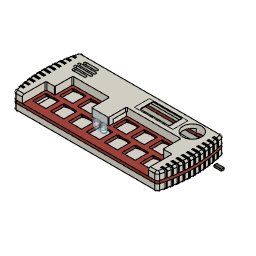
pianissimo_retro_case (Autodesk Fusion 360 design; units mm, degrees)
Autodesk Fusion 360 part; units mm, degrees
(part 1 of 2)
sketch "acrylic_import" plane through (0, 0, 0) normal (0, 0, 1) x (1, 0, 0)
  line L0 (-9.525, 176.95625) -> (51.15, 176.95625)
  line L1 (51.15, 171.95625) -> (51.15, 176.95625)
  line L2 (21.5, 189.35) -> (35.65, 189.35)
  line L3 (63.15, 171.95625) -> (63.15, 176.95625)
  line L4 (116.75, 189.35) -> (130.9, 189.35)
  line L5 (63.15, 171.95625) -> (133.875, 171.95625)
  circle A0 centre (-5.025, 185.875) radius 1.5
  line L6 (63.15, 176.95625) -> (142.875, 176.95625)
  circle A1 centre (-5.025, 172.45625) radius 1.5
  line L7 (133.875, 171.95625) -> (133.875, 111.375)
  line L8 (-0.525, 111.375) -> (133.875, 111.375)
  line L9 (-9.525, 101.95625) -> (-9.525, 31.375)
  circle A2 centre (-5.025, 35.875) radius 1.5
  circle A3 centre (138.375, 185.875) radius 1.5
  line L10 (-9.525, 106.375) -> (142.875, 106.375)
  line L11 (142.875, 101.95625) -> (142.875, 31.375)
  line L12 (59.6, 189.35) -> (73.75, 189.35)
  line L13 (142.875, 106.375) -> (142.875, 176.95625)
  line L14 (-9.525, 176.95625) -> (-9.525, 106.375)
  circle A4 centre (-5.025, 97.45625) radius 1.5
  line L15 (40.55, 189.35) -> (54.7, 189.35)
  line L16 (142.875, -43.625) -> (142.875, 26.95625)
  line L17 (35.65, 189.35) -> (35.65, 203.5)
  circle A5 centre (138.375, 172.45625) radius 1.5
  line L18 (63.15, 96.95625) -> (63.15, 101.95625)
  line L19 (2.45, 189.35) -> (16.6, 189.35)
  line L20 (-0.525, 111.375) -> (-0.525, 171.95625)
  line L21 (97.7, 189.35) -> (111.85, 189.35)
  line L22 (-0.525, 171.95625) -> (51.15, 171.95625)
  circle A6 centre (138.375, 110.875) radius 1.5
  line L23 (142.875, 101.95625) -> (63.15, 101.95625)
  circle A7 centre (-5.025, -39.125) radius 1
  circle A8 centre (-5.025, 22.45625) radius 1
  line L24 (-9.525, 251.95625) -> (-9.525, 181.375)
  line L25 (-9.525, 181.375) -> (142.875, 181.375)
  circle A9 centre (-5.025, 110.875) radius 1.5
  line L26 (78.65, 189.35) -> (92.8, 189.35)
  line L27 (-9.525, -43.625) -> (142.875, -43.625)
  line L28 (111.85, 189.35) -> (111.85, 203.5)
  line L29 (78.65, 203.5) -> (78.65, 189.35)
  circle A10 centre (138.375, 22.45625) radius 1
  line L30 (-9.525, 26.95625) -> (142.875, 26.95625)
  circle A11 centre (138.375, 97.45625) radius 1.5
  line L31 (133.875, 36.375) -> (133.875, 96.95625)
  line L32 (51.15, 96.95625) -> (51.15, 101.95625)
  line L33 (59.6, 203.5) -> (59.6, 189.35)
  line L34 (-9.525, 101.95625) -> (51.15, 101.95625)
  circle A12 centre (138.375, -39.125) radius 1
  line L35 (-9.525, 26.95625) -> (-9.525, -43.625)
  line L36 (-0.525, 36.375) -> (133.875, 36.375)
  line L37 (51.15, 96.95625) -> (-0.525, 96.95625)
  line L38 (-9.525, 31.375) -> (142.875, 31.375)
  circle A13 centre (138.375, 35.875) radius 1.5
  line L39 (-0.525, 96.95625) -> (-0.525, 36.375)
  line L40 (63.15, 96.95625) -> (133.875, 96.95625)
  arc A14 (120.930314, 228.525) -> (126.719686, 228.525) centre (123.825, 238.096875) ccw
  arc A15 (128.463046, 246.95625) -> (119.186954, 246.95625) centre (123.825, 238.096875) ccw
  line L41 (88.175, 208.4) -> (102.325, 208.4)
  line L42 (16.6, 189.35) -> (16.6, 203.5)
  line L43 (63.15, 246.95625) -> (63.15, 251.95625)
  line L44 (83.275, 208.4) -> (83.275, 222.55)
  circle A16 centre (138.375, 247.45625) radius 1.5
  line L45 (111.85, 203.5) -> (97.7, 203.5)
  circle A17 centre (138.375, 260.875) radius 1.5
  line L46 (2.45, 203.5) -> (2.45, 189.35)
  line L47 (133.875, 228.525) -> (133.875, 246.95625)
  line L48 (102.325, 208.4) -> (102.325, 222.55)
  line L49 (69.125, 208.4) -> (83.275, 208.4)
  line L50 (63.15, 251.95625) -> (142.875, 251.95625)
  line L51 (133.875, 228.525) -> (126.719686, 228.525)
  line L52 (130.9, 203.5) -> (116.75, 203.5)
  line L53 (92.8, 203.5) -> (78.65, 203.5)
  line L54 (102.325, 222.55) -> (88.175, 222.55)
  line L55 (83.275, 222.55) -> (69.125, 222.55)
  line L56 (121.375, 208.4) -> (121.375, 222.55)
  line L57 (121.375, 222.55) -> (107.225, 222.55)
  line L58 (107.225, 208.4) -> (121.375, 208.4)
  line L59 (69.125, 222.55) -> (69.125, 208.4)
  line L60 (88.175, 222.55) -> (88.175, 208.4)
  line L61 (107.225, 222.55) -> (107.225, 208.4)
  arc A18 (3.381227, 395.390581) -> (3.386093, 392.890586) centre (3.38366, 394.140584) ccw
  line L62 (9, 281.475) -> (9, 300.525)
  arc A19 (15.876065, 392.914896) -> (15.871199, 395.414891) centre (15.873632, 394.164893) ccw
  line L63 (9, 375.525) -> (48.15, 375.525)
  line L64 (-9.525, 401.95625) -> (-9.525, 331.375)
  line L65 (15.876065, 392.914896) -> (3.386093, 392.890586)
  line L66 (9, 356.475) -> (9, 375.525)
  line L67 (-0.525, 281.475) -> (9, 281.475)
  line L68 (48.15, 300.525) -> (48.15, 303.525)
  line L69 (1.169417, 391.395696) -> (18.021701, 391.414893)
  line L70 (-0.525, 331.375) -> (-0.525, 356.475)
  circle A20 centre (-5.025, 335.875) radius 1
  circle A21 centre (-5.025, 322.45625) radius 1.5
  circle A22 centre (-5.025, 397.45625) radius 1
  arc A23 (18.024549, 388.914894) -> (18.021701, 391.414893) centre (18.023125, 390.164893) ccw
  arc A24 (18.024544, 384.914894) -> (18.021707, 387.414893) centre (18.023125, 386.164893) ccw
  line L71 (15.877503, 380.914899) -> (3.387616, 380.876226)
  line L72 (18.024544, 384.914894) -> (1.172264, 384.895769)
  line L73 (-9.525, 331.375) -> (-0.525, 331.375)
  line L74 (48.15, 356.475) -> (48.15, 375.525)
  line L75 (3.379875, 383.376214) -> (15.869762, 383.414887)
  line L76 (3.381227, 395.390581) -> (15.871199, 395.414891)
  arc A25 (1.169417, 391.395696) -> (1.172265, 388.895698) centre (1.170841, 390.145697) ccw
  line L77 (133.875, 356.475) -> (133.875, 331.375)
  line L78 (133.875, 356.475) -> (124.35, 356.475)
  line L79 (1.169426, 387.395767) -> (18.021707, 387.414893)
  line L80 (9, 300.525) -> (48.15, 300.525)
  line L81 (48.15, 303.525) -> (-0.525, 303.525)
  arc A26 (15.877503, 380.914899) -> (15.869762, 383.414887) centre (15.873632, 382.164893) ccw
  line L82 (18.024549, 388.914894) -> (1.172265, 388.895698)
  arc A27 (3.379875, 383.376214) -> (3.387616, 380.876226) centre (3.383745, 382.12622) ccw
  line L83 (48.15, 211.475) -> (48.15, 225.525)
  line L84 (97.7, 203.5) -> (97.7, 189.35)
  circle A28 centre (-5.025, 260.875) radius 1.5
  arc A29 (142.875, 181.375) -> (142.875, 251.95625) centre (20.832179, 216.665625) ccw
  line L85 (63.15, 246.95625) -> (119.186954, 246.95625)
  line L86 (66.15, 225.525) -> (66.15, 211.475)
  line L87 (66.15, 225.525) -> (66.15, 228.525)
  line L88 (120.930314, 228.525) -> (66.15, 228.525)
  line L89 (73.75, 189.35) -> (73.75, 203.5)
  line L90 (40.55, 203.5) -> (40.55, 189.35)
  line L91 (54.7, 189.35) -> (54.7, 203.5)
  line L92 (128.463046, 246.95625) -> (133.875, 246.95625)
  line L93 (133.875, 256.375) -> (142.875, 256.375)
  line L94 (54.7, 203.5) -> (40.55, 203.5)
  line L95 (-0.525, 246.95625) -> (51.15, 246.95625)
  line L96 (119.186954, 321.95625) -> (-0.525, 321.95625)
  line L97 (66.15, 211.475) -> (48.15, 211.475)
  line L98 (73.75, 203.5) -> (59.6, 203.5)
  line L99 (-0.525, 246.95625) -> (-0.525, 228.525)
  line L100 (-9.525, 251.95625) -> (51.15, 251.95625)
  circle A30 centre (-5.025, 247.45625) radius 1.5
  line L101 (133.875, 281.475) -> (133.875, 256.375)
  line L102 (45.175, 208.4) -> (45.175, 222.55)
  line L103 (142.875, 256.375) -> (142.875, 326.95625)
  line L104 (26.125, 222.55) -> (11.975, 222.55)
  line L105 (11.975, 208.4) -> (26.125, 208.4)
  line L106 (35.65, 203.5) -> (21.5, 203.5)
  arc A31 (-9.525, 251.95625) -> (-9.525, 181.375) centre (112.517821, 216.665625) ccw
  line L107 (130.9, 189.35) -> (130.9, 203.5)
  line L108 (116.75, 203.5) -> (116.75, 189.35)
  line L109 (-9.525, 326.95625) -> (-9.525, 256.375)
  line L110 (31.025, 222.55) -> (31.025, 208.4)
  line L111 (66.15, 356.475) -> (48.15, 356.475)
  line L112 (21.5, 203.5) -> (21.5, 189.35)
  line L113 (142.875, 181.375) -> (142.875, 251.95625)
  line L114 (-9.525, 256.375) -> (-0.525, 256.375)
  line L115 (-0.525, 256.375) -> (-0.525, 281.475)
  line L116 (51.15, 246.95625) -> (51.15, 251.95625)
  line L117 (-9.525, 326.95625) -> (142.875, 326.95625)
  line L118 (45.175, 222.55) -> (31.025, 222.55)
  line L119 (92.8, 189.35) -> (92.8, 203.5)
  line L120 (16.6, 203.5) -> (2.45, 203.5)
  line L121 (11.975, 222.55) -> (11.975, 208.4)
  line L122 (26.125, 208.4) -> (26.125, 222.55)
  line L123 (31.025, 208.4) -> (45.175, 208.4)
  circle A32 centre (138.375, 397.45625) radius 1
  line L124 (48.15, 228.525) -> (-0.525, 228.525)
  line L125 (124.35, 375.525) -> (66.15, 375.525)
  line L126 (142.875, 331.375) -> (142.875, 401.95625)
  line L127 (124.35, 356.475) -> (124.35, 375.525)
  line L128 (133.875, 331.375) -> (142.875, 331.375)
  line L129 (-9.525, 401.95625) -> (142.875, 401.95625)
  line L130 (-0.525, 356.475) -> (9, 356.475)
  line L131 (66.15, 300.525) -> (66.15, 303.525)
  line L132 (128.463046, 321.95625) -> (133.875, 321.95625)
  circle A33 centre (138.375, 322.45625) radius 1.5
  line L133 (66.15, 375.525) -> (66.15, 356.475)
  line L134 (124.35, 281.475) -> (124.35, 300.525)
  line L135 (48.15, 225.525) -> (48.15, 228.525)
  line L136 (133.875, 303.525) -> (133.875, 321.95625)
  line L137 (133.875, 281.475) -> (124.35, 281.475)
  line L138 (133.875, 303.525) -> (126.719686, 303.525)
  line L139 (-0.525, 321.95625) -> (-0.525, 303.525)
  line L140 (120.930314, 303.525) -> (66.15, 303.525)
  circle A34 centre (138.375, 335.875) radius 1
  arc A35 (1.169426, 387.395767) -> (1.172264, 384.895768) centre (1.170845, 386.145768) ccw
  arc A36 (128.463046, 321.95625) -> (119.186954, 321.95625) centre (123.825, 313.096875) ccw
  circle A37 centre (123.825, 388.096875) radius 10
  line L141 (124.35, 300.525) -> (66.15, 300.525)
  arc A38 (120.930314, 303.525) -> (126.719686, 303.525) centre (123.825, 313.096875) ccw
  point P0 (-5.025, 172.45625)
  dimension "d157" = 2
  dimension "d158" = 2
  dimension "d159" = 2
  dimension "d160" = 2
  dimension "d161" = 3
  dimension "d162" = 3
  dimension "d163" = 3
  dimension "d164" = 3
  dimension "d165" = 3
  dimension "d166" = 3
  dimension "d167" = 3
  dimension "d168" = 3
  dimension "d169" = 3
  dimension "d170" = 3
  dimension "d171" = 3
  dimension "d172" = 3
  dimension "d173" = 3
  dimension "d174" = 3
  dimension "d175" = 3
  dimension "d176" = 2
  dimension "d177" = 2
  dimension "d178" = 2
  dimension "d179" = 2
  dimension "d180" = 3
  dimension "d181" = 20
  dimension "d182" = 2.5
  dimension "d183" = 2.5
  dimension "d184" = 2.5
  dimension "d185" = 2.5
  dimension "d186" = 2.5
  dimension "d187" = 2.5
  dimension "d188" = 2.5
  dimension "d189" = 2.5
  dimension "d190" = 20
  dimension "d191" = 20
  constraint perpendicular L51 L99
  constraint coincident L124.start L51
  constraint perpendicular L51 L135
  constraint perpendicular L51 L87
  constraint perpendicular L47 L95
  constraint perpendicular L138 L139
  constraint coincident L68.end L138
  constraint perpendicular L68 L138
  constraint perpendicular L131 L138
  constraint coincident L93.start L114
  constraint perpendicular L111 L133
  constraint coincident L77.end L73
  constraint collinear L0 L6
  constraint collinear L5 L22
  constraint collinear L50 L100
  constraint collinear L85 L95
  constraint collinear L51 L124
  constraint collinear L93 L114
  constraint collinear L81 L138
  constraint collinear L73 L128
  constraint perpendicular L27 L35
  constraint perpendicular L16 L30
  constraint perpendicular L64 L73
  constraint perpendicular L70 L130
  constraint perpendicular L126 L129
  constraint perpendicular L77 L128
  constraint perpendicular L109 L114
  constraint perpendicular L67 L115
  constraint perpendicular L93 L101
  constraint perpendicular L24 L25
  constraint perpendicular L25 L113
  constraint perpendicular L10 L14
  constraint perpendicular L6 L13
  constraint perpendicular L7 L8
  constraint perpendicular L20 L22
  constraint perpendicular L36 L39
  constraint perpendicular L9 L38
  constraint tangent A18 L76
  constraint tangent A19 L76
  constraint tangent A19 L65
  constraint tangent A18 L65
  constraint tangent L69 A25
  constraint tangent L69 A23
  constraint tangent A23 L82
  constraint tangent A25 L82
  constraint tangent L79 A35
  constraint tangent A24 L79
  constraint tangent A24 L72
  constraint tangent L72 A35
  constraint tangent L75 A27
  constraint tangent L75 A26
  constraint tangent L71 A26
  constraint tangent L71 A27
  constraint collinear L85 L92
  constraint collinear L51 L88
  constraint concentric A14 A15
  constraint collinear L138 L140
  constraint concentric A36 A38
  constraint perpendicular L103 L117
  constraint perpendicular L96 L139
  constraint perpendicular L32 L34
  constraint perpendicular L37 L39
  constraint perpendicular L31 L40
  constraint perpendicular L18 L23
  measures "d157" diameter of A7
  measures "d158" diameter of A8
  measures "d159" diameter of A10
  measures "d160" diameter of A12
  measures "d161" diameter of A2
  measures "d162" diameter of A4
  measures "d163" diameter of A11
  measures "d164" diameter of A13
  measures "d165" diameter of A9
  measures "d166" diameter of A5
  measures "d167" diameter of A6
  measures "d168" diameter of A0
  measures "d169" diameter of A30
  measures "d170" diameter of A16
  measures "d171" diameter of A3
  measures "d172" diameter of A1
  measures "d173" diameter of A28
  measures "d174" diameter of A33
  measures "d175" diameter of A17
  measures "d176" diameter of A20
  measures "d177" diameter of A22
  measures "d178" diameter of A32
  measures "d179" diameter of A34
  measures "d180" diameter of A21
  measures "d181" diameter of A37
  measures "d182" diameter of A19
  measures "d183" diameter of A23
  measures "d184" diameter of A24
  measures "d185" diameter of A26
  measures "d186" diameter of A27
  measures "d187" diameter of A35
  measures "d188" diameter of A25
  measures "d189" diameter of A18
  measures "d190" diameter of A36
  measures "d191" diameter of A15
sketch "plate" plane through (0, 0, 0) normal (0, 0, 1) x (1, 0, 0)
  line L0 (111.85, -21.5) -> (97.7, -21.5)
  line L1 (121.375, -2.45) -> (107.225, -2.45)
  line L2 (88.175, -16.6) -> (102.325, -16.6)
  line L3 (83.275, -16.6) -> (83.275, -2.45)
  line L4 (102.325, -16.6) -> (102.325, -2.45)
  line L5 (83.275, -2.45) -> (69.125, -2.45)
  line L6 (130.9, -21.5) -> (116.75, -21.5)
  line L7 (69.125, -2.45) -> (69.125, -16.6)
  line L8 (107.225, -2.45) -> (107.225, -16.6)
  line L9 (88.175, -2.45) -> (88.175, -16.6)
  line L10 (102.325, -2.45) -> (88.175, -2.45)
  line L11 (121.375, -16.6) -> (121.375, -2.45)
  line L12 (92.8, -21.5) -> (78.65, -21.5)
  line L13 (120.930314, 3.525) -> (66.65, 3.525)
  line L14 (92.8, -35.65) -> (92.8, -21.5)
  line L15 (130.9, -35.65) -> (130.9, -21.5)
  line L16 (73.75, -35.65) -> (73.75, -21.5)
  line L17 (63.15, 21.95625) -> (63.15, 26.95625)
  line L18 (128.463046, 21.95625) -> (133.875, 21.95625)
  line L19 (116.75, -21.5) -> (116.75, -35.65)
  arc A0 (128.463046, 21.95625) -> (119.186954, 21.95625) centre (123.825, 13.096875) ccw
  line L20 (66.65, 0.525) -> (66.65, -13.525)
  line L21 (69.125, -16.6) -> (83.275, -16.6)
  line L22 (16.6, -35.65) -> (16.6, -21.5)
  line L23 (107.225, -16.6) -> (121.375, -16.6)
  line L24 (142.875, -43.625) -> (142.875, 26.95625)
  line L25 (-9.525, 26.95625) -> (-9.525, -43.625)
  line L26 (63.15, 21.95625) -> (119.186954, 21.95625)
  line L27 (97.7, -21.5) -> (97.7, -35.772243)
  line L28 (133.875, 3.525) -> (126.719686, 3.525)
  line L29 (133.875, 3.525) -> (133.875, 21.95625)
  arc A1 (120.930314, 3.525) -> (126.719686, 3.525) centre (123.825, 13.096875) ccw
  line L30 (21.5, -21.5) -> (21.5, -35.65)
  line L31 (63.15, 26.95625) -> (142.875, 26.95625)
  line L32 (111.85, -35.772243) -> (111.85, -21.5)
  line L33 (35.65, -35.65) -> (35.65, -21.5)
  circle A2 centre (138.375, 22.45625) radius 1.05
  line L34 (66.65, 0.525) -> (66.65, 3.525)
  line L35 (54.7, -35.65) -> (54.7, -21.5)
  line L36 (26.125, -2.45) -> (11.975, -2.45)
  line L37 (97.7, -35.772243) -> (111.85, -35.772243)
  line L38 (40.55, -21.5) -> (40.55, -35.65)
  line L39 (-9.525, 26.95625) -> (51.15, 26.95625)
  line L40 (31.025, -16.6) -> (45.175, -16.6)
  line L41 (78.65, -21.5) -> (78.65, -35.65)
  line L42 (59.6, -21.5) -> (59.6, -35.65)
  line L43 (47.65, 3.525) -> (-0.525, 3.525)
  line L44 (47.65, -13.525) -> (47.65, 0.525)
  line L45 (40.55, -35.65) -> (54.7, -35.65)
  line L46 (45.175, -2.45) -> (31.025, -2.45)
  arc A3 (-9.525, 26.95625) -> (-9.525, -43.625) centre (112.517821, -8.334375) ccw
  circle A4 centre (-5.025, -39.125) radius 1.05
  line L47 (-9.525, -43.625) -> (142.875, -43.625)
  line L48 (16.6, -21.5) -> (2.45, -21.5)
  line L49 (-0.525, 21.95625) -> (51.15, 21.95625)
  line L50 (35.65, -21.5) -> (21.5, -21.5)
  line L51 (-0.525, 21.95625) -> (-0.525, 3.525)
  circle A5 centre (-5.025, 22.45625) radius 1.05
  line L52 (73.75, -21.5) -> (59.6, -21.5)
  line L53 (31.025, -2.45) -> (31.025, -16.6)
  arc A6 (142.875, -43.625) -> (142.875, 26.95625) centre (20.832179, -8.334375) ccw
  line L54 (47.65, 0.525) -> (47.65, 3.525)
  line L55 (21.5, -35.65) -> (35.65, -35.65)
  line L56 (11.975, -2.45) -> (11.975, -16.6)
  line L57 (11.975, -16.6) -> (26.125, -16.6)
  line L58 (116.75, -35.65) -> (130.9, -35.65)
  line L59 (78.65, -35.65) -> (92.8, -35.65)
  line L60 (26.125, -16.6) -> (26.125, -2.45)
  line L61 (66.65, -13.525) -> (47.65, -13.525)
  line L62 (54.7, -21.5) -> (40.55, -21.5)
  line L63 (51.15, 21.95625) -> (51.15, 26.95625)
  line L64 (59.6, -35.65) -> (73.75, -35.65)
  circle A7 centre (138.375, -39.125) radius 1.05
  line L65 (45.175, -16.6) -> (45.175, -2.45)
  line L66 (2.45, -21.5) -> (2.45, -35.65)
  line L67 (2.45, -35.65) -> (16.6, -35.65)
  line L68 (51.15, 26.95625) -> (63.15, 26.95625)
  line L69 (63.15, 21.95625) -> (51.15, 21.95625)
  line L70 (46.15, 23.95625) -> (46.15, 24.95625)
  line L71 (41.65, 23.95625) -> (41.65, 24.95625)
  line L72 (68.15, 23.95625) -> (68.15, 24.95625)
  line L73 (72.65, 23.95625) -> (72.65, 24.95625)
  line L74 (42.15, 25.45625) -> (45.65, 25.45625)
  line L75 (42.15, 23.45625) -> (45.65, 23.45625)
  line L76 (68.65, 25.45625) -> (72.15, 25.45625)
  line L77 (68.65, 23.45625) -> (72.15, 23.45625)
  arc A8 (42.15, 25.45625) -> (41.65, 24.95625) centre (42.15, 24.95625) ccw
  arc A9 (41.65, 23.95625) -> (42.15, 23.45625) centre (42.15, 23.95625) ccw
  arc A10 (45.65, 23.45625) -> (46.15, 23.95625) centre (45.65, 23.95625) ccw
  arc A11 (46.15, 24.95625) -> (45.65, 25.45625) centre (45.65, 24.95625) ccw
  arc A12 (68.65, 25.45625) -> (68.15, 24.95625) centre (68.65, 24.95625) ccw
  arc A13 (72.65, 24.95625) -> (72.15, 25.45625) centre (72.15, 24.95625) ccw
  arc A14 (72.15, 23.45625) -> (72.65, 23.95625) centre (72.15, 23.95625) ccw
  arc A15 (68.15, 23.95625) -> (68.65, 23.45625) centre (68.65, 23.95625) ccw
  line L78 (160.000002, 0) -> (168.000002, 0)
  line L79 (168.000002, 0) -> (168.000002, 3)
  line L80 (168.000002, 3) -> (160.000002, 3)
  line L81 (160.000002, 3) -> (160.000002, 0)
  dimension "d36" = 2.1
  dimension "d37" = 2.1
  dimension "d38" = 2.1
  dimension "d39" = 2.1
  dimension "d40" = 20
  dimension "d216" = 0.5
  dimension "d220" = 8
  dimension "d221" = 3
  constraint perpendicular L28 L51
  constraint coincident L43.start L28
  constraint perpendicular L28 L54
  constraint perpendicular L28 L34
  constraint perpendicular L29 L49
  constraint collinear L31 L39
  constraint collinear L26 L49
  constraint collinear L28 L43
  constraint perpendicular L25 L47
  constraint perpendicular L24 L47
  constraint collinear L18 L26
  constraint collinear L13 L28
  constraint concentric A0 A1
  constraint perpendicular L17 L68
  constraint perpendicular L63 L69
  constraint tangent L76 A12
  constraint tangent L72 A12
  constraint tangent L76 A13
  constraint tangent L77 A14
  constraint tangent L77 A15
  constraint tangent L72 A15
  constraint horizontal L78
  constraint vertical L79
  constraint horizontal L80
  constraint vertical L81
  measures "d36" diameter of A4
  measures "d37" diameter of A5
  measures "d38" diameter of A2
  measures "d39" diameter of A7
  measures "d40" diameter of A0
  measures "d216" radius of A8
sketch "bottom" plane through (0, 0, 0) normal (0, 0, 1) x (1, 0, 0)
  line L0 (-9.525, 26.95625) -> (-9.525, -43.625)
  line L1 (-9.525, -43.625) -> (142.875, -43.625)
  circle A0 centre (138.375, 22.45625) radius 2.5
  circle A1 centre (-5.025, 22.45625) radius 2.5
  line L2 (-0.525, -38.625) -> (133.875, -38.625)
  circle A2 centre (-5.025, -39.125) radius 2.5
  line L3 (133.875, -38.625) -> (133.875, 21.95625)
  circle A3 centre (138.375, -39.125) radius 2.5
  line L4 (51.15, 21.95625) -> (51.15, 26.95625)
  line L5 (142.875, 26.95625) -> (142.875, -43.625)
  line L6 (-0.525, 21.95625) -> (-0.525, -38.625)
  line L7 (63.15, 21.95625) -> (63.15, 26.95625)
  arc A4 (142.875, -43.625) -> (142.875, 26.95625) centre (20.832179, -8.334375) ccw
  arc A5 (-9.525, 26.95625) -> (-9.525, -43.625) centre (112.517821, -8.334375) ccw
  line L8 (-0.525, 21.95625) -> (133.875, 21.95625)
  line L9 (-9.525, 26.95625) -> (142.875, 26.95625)
  circle A6 centre (-5.025, 22.45625) radius 1.05
  circle A7 centre (138.375, 22.45625) radius 1.05
  circle A8 centre (138.375, -39.125) radius 1.05
  circle A9 centre (-5.025, -39.125) radius 1.05
  dimension "d41" = 5
  dimension "d42" = 5
  dimension "d43" = 5
  dimension "d44" = 5
  dimension "d195" = 2.1
  dimension "d196" = 2.1
  dimension "d197" = 2.1
  dimension "d198" = 2.1
  constraint perpendicular L2 L6
  constraint perpendicular L0 L1
  constraint perpendicular L3 L8
  constraint perpendicular L0 L9
  constraint concentric A1 A6
  constraint concentric A0 A7
  constraint concentric A3 A8
  constraint concentric A2 A9
  measures "d41" diameter of A2
  measures "d42" diameter of A1
  measures "d43" diameter of A0
  measures "d44" diameter of A3
  measures "d195" diameter of A6
  measures "d196" diameter of A7
  measures "d197" diameter of A8
  measures "d198" diameter of A9
sketch "top" plane through (0, 0, 0) normal (0, 0, 1) x (1, 0, 0)
  line L0 (133.875, -43.625) -> (142.875, -43.625)
  line L1 (124.35, 0.525) -> (66.15, 0.525)
  line L2 (124.35, -18.525) -> (124.35, 0.525)
  line L3 (66.15, 0.525) -> (66.15, -18.525)
  line L4 (133.875, -18.525) -> (133.875, -43.625)
  line L5 (48.15, -18.525) -> (48.15, 0.525)
  line L6 (-9.525, 26.95625) -> (142.875, 26.95625)
  circle A0 centre (138.375, 22.45625) radius 1.5
  line L7 (-9.525, 26.95625) -> (-9.525, -43.625)
  line L8 (66.15, -18.525) -> (48.15, -18.525)
  line L9 (133.875, -18.525) -> (124.35, -18.525)
  circle A1 centre (-5.025, -39.125) radius 1.5
  line L10 (142.875, -43.625) -> (142.875, 26.95625)
  circle A2 centre (138.375, -39.125) radius 1.5
  circle A3 centre (-5.025, 22.45625) radius 1.5
  line L11 (9, -18.525) -> (9, 0.525)
  line L12 (-0.525, -43.625) -> (-0.525, -18.525)
  line L13 (-0.525, -18.525) -> (9, -18.525)
  line L14 (9, 0.525) -> (48.15, 0.525)
  line L15 (-9.525, -43.625) -> (-0.525, -43.625)
  line L16 (48.15, 3.525) -> (-0.525, 3.525)
  line L17 (48.15, 0.525) -> (48.15, 3.525)
  line L18 (66.15, 0.525) -> (66.15, 3.525)
  line L19 (66.15, 3.525) -> (133.875, 3.525)
  line L20 (133.875, 3.525) -> (133.875, 21.95625)
  line L21 (-0.525, 21.95625) -> (133.875, 21.95625)
  line L22 (-0.525, 21.95625) -> (-0.525, 3.525)
  arc A4 (-9.525, 26.95625) -> (-9.525, -43.625) centre (112.517821, -8.334375) ccw
  arc A5 (142.875, -43.625) -> (142.875, 26.95625) centre (20.832179, -8.334375) ccw
  line L23 (66.15, -13.525) -> (48.15, -13.525)
  dimension "d49" = 3
  dimension "d50" = 3
  dimension "d51" = 3
  dimension "d56" = 3
  constraint perpendicular L3 L8
  constraint coincident L0.start L15
  constraint collinear L0 L15
  constraint perpendicular L7 L15
  constraint perpendicular L12 L13
  constraint perpendicular L6 L10
  constraint perpendicular L0 L4
  constraint perpendicular L19 L20
  constraint perpendicular L20 L21
  measures "d49" diameter of A1
  measures "d50" diameter of A0
  measures "d51" diameter of A2
  measures "d56" diameter of A3
sketch "top_holes" plane through (0, 0, 0) normal (0, 0, 1) x (1, 0, 0)
  arc A0 (3.379875, 8.376214) -> (3.387616, 5.876226) centre (3.383745, 7.12622) ccw
  line L0 (3.379875, 8.376214) -> (15.869762, 8.414887)
  arc A1 (15.877503, 5.914899) -> (15.869762, 8.414887) centre (15.873632, 7.164893) ccw
  line L1 (15.877503, 5.914899) -> (3.387616, 5.876226)
  arc A2 (1.169426, 12.395767) -> (1.172264, 9.895768) centre (1.170845, 11.145768) ccw
  line L2 (1.169426, 12.395767) -> (18.021707, 12.414893)
  arc A3 (18.024544, 9.914894) -> (18.021707, 12.414893) centre (18.023125, 11.164893) ccw
  line L3 (18.024544, 9.914894) -> (1.172264, 9.895769)
  arc A4 (1.169417, 16.395696) -> (1.172265, 13.895698) centre (1.170841, 15.145697) ccw
  line L4 (1.169417, 16.395696) -> (18.021701, 16.414893)
  arc A5 (18.024549, 13.914894) -> (18.021701, 16.414893) centre (18.023125, 15.164893) ccw
  line L5 (18.024549, 13.914894) -> (1.172265, 13.895698)
  arc A6 (3.381227, 20.390581) -> (3.386093, 17.890586) centre (3.38366, 19.140584) ccw
  line L6 (3.381227, 20.390581) -> (15.871199, 20.414891)
  arc A7 (15.876065, 17.914896) -> (15.871199, 20.414891) centre (15.873632, 19.164893) ccw
  line L7 (15.876065, 17.914896) -> (3.386093, 17.890586)
  circle A8 centre (123.825, 13.096875) radius 10
  dimension "d67" = 20
  dimension "d68" = 2.5
  dimension "d69" = 2.5
  dimension "d70" = 2.5
  dimension "d71" = 2.5
  dimension "d72" = 2.5
  dimension "d73" = 2.5
  dimension "d74" = 2.5
  dimension "d75" = 2.5
  constraint tangent A6 L6
  constraint tangent L6 A7
  constraint tangent A7 L7
  constraint tangent A6 L7
  constraint tangent A4 L4
  constraint tangent L4 A5
  constraint tangent A5 L5
  constraint tangent A4 L5
  constraint tangent A2 L2
  constraint tangent L2 A3
  constraint tangent A3 L3
  constraint tangent A2 L3
  constraint tangent A0 L0
  constraint tangent L0 A1
  constraint tangent A1 L1
  constraint tangent A0 L1
  measures "d67" diameter of A8
  measures "d68" diameter of A7
  measures "d69" diameter of A5
  measures "d70" diameter of A3
  measures "d71" diameter of A1
  measures "d72" diameter of A0
  measures "d73" diameter of A2
  measures "d74" diameter of A4
  measures "d75" diameter of A6
extrude "Extrude1" add sketch "plate" against normal blind 3 contours L13 L17 L18 A0 L20 L24 L25 L26 L28 L29 A1 L31 L34 L39 L43 L44 L47 L49 L51 L54 L61 L63 | L17 L63 L68 L69 | L24 A6 | L25 A3 | A2 | A4 | A5 | A7 | L70 L71 L74 L75 A8 A9 A10 A11 | L72 L73 L76 L77 A12 A13 A14 A15 picked at (4.633333, -6.808333) picked at (59.15, 23.622917) picked at (144.12293, -14.274886) picked at (-10.77293, -2.393864) picked at (138.452882, 23.273596) picked at (-4.735816, -39.322162) picked at (-4.939523, 22.339037) picked at (138.297118, -39.942346) picked at (44.483333, 24.122917) picked at (69.816667, 24.122917) makes body 1
extrude "Extrude2" add sketch "top" along normal blind 8 separate body contours L0 L1 L2 L4 L6 L7 L9 L10 L11 L12 L13 L14 L15 L16 L17 L18 L19 L20 L21 L22 | L10 A5 | L7 A4 | L3 L5 L16 L17 L18 L19 L20 L21 L22 L23 | L3 L5 L8 L23 | A0 | A1 | A2 | A3 picked at (-6.525, -11.73125) picked at (144.12293, -14.274886) picked at (-10.77293, -2.393864) picked at (60.5, 15.8125) picked at (54.15, -15.191667) picked at (138.047024, 22.954852) picked at (-5.685457, -38.762887) picked at (138.48626, -39.612464) picked at (-5.495036, 21.990072) makes body 2
extrude "Extrude3" add sketch "bottom" against normal blind 8 from surface at -3 separate body contours L0 L1 L2 L3 L4 L5 L6 L7 L8 L9 | L0 A5 | L4 L7 L8 L9 | L5 A4 | L2 L3 L6 L8 | A0 | A1 | A2 | A3 | A6 | A7 | A8 | A9 picked at (86.725, 23.622917) picked at (-10.77293, -14.274886) picked at (55.15, 25.289583) picked at (144.12293, -14.274886) picked at (65.5, -18.43125) picked at (137.757246, 20.542276) picked at (-3.02155, 22.279883) picked at (-3.017641, -39.249202) picked at (137.757246, -41.038974) picked at (-4.939523, 22.339037) picked at (138.452882, 21.638904) picked at (138.297118, -38.307654) picked at (-4.735816, -39.322162) makes body 3
extrude "Extrude4" cut sketch "top" along normal blind 4 contours L3 L5 L16 L17 L18 L19 L20 L21 L22 L23 picked at (60.5, 15.8125) bodies 2
extrude "Extrude5" cut sketch "top_holes" along normal up to surface (8 mm away) contours A0 L0 A1 L1 | A2 L2 A3 L3 | A4 L4 A5 L5 | A6 L6 A7 L7 | A8 picked at (11.709046, 7.568667) picked at (6.788745, 10.735476) picked at (6.788744, 14.735429) picked at (11.711119, 18.740124) picked at (128.408328, 10.501234) bodies 2
extrude "Extrude6" cut sketch "bottom" against normal blind 9 contours L2 L3 L6 L8 picked at (65.5, -18.43125) bodies 3
sketch "sink" plane through (0, 0, 0) normal (0, 0, 1) x (1, 0, 0)
  line L0 (-13.521064, -7.334375) -> (-28, -7.334375)
  line L1 (66.675, 35.245101) -> (66.675, -62.292438)
  line L2 (-13.521064, -9.334375) -> (-28, -9.334375)
  line L3 (-10.730432, -34.834375) -> (-28, -34.834375)
  line L4 (-10.286978, -36.834375) -> (-30, -36.834375)
  line L5 (-11.777344, -29.334375) -> (-28, -29.334375)
  line L6 (-11.42568, -31.334375) -> (-28, -31.334375)
  line L7 (-12.575908, -23.834375) -> (-28, -23.834375)
  line L8 (-12.313925, -25.834375) -> (-28, -25.834375)
  line L9 (-13.13082, -18.334375) -> (-28, -18.334375)
  line L10 (-12.956992, -20.334375) -> (-28, -20.334375)
  line L11 (-13.445277, -12.834375) -> (-28, -12.834375)
  line L12 (-13.358609, -14.834375) -> (-28, -14.834375)
  line L13 (-13.358609, -1.834375) -> (-28, -1.834375)
  line L14 (-13.445277, -3.834375) -> (-28, -3.834375)
  line L15 (-12.956992, 3.665625) -> (-28, 3.665625)
  line L16 (-13.13082, 1.665625) -> (-28, 1.665625)
  line L17 (-12.313925, 9.165625) -> (-28, 9.165625)
  line L18 (-12.575908, 7.165625) -> (-28, 7.165625)
  line L19 (-11.42568, 14.665625) -> (-28, 14.665625)
  line L20 (-11.777344, 12.665625) -> (-28, 12.665625)
  line L21 (-10.286978, 20.165625) -> (-30, 20.165625)
  line L22 (-10.730432, 18.165625) -> (-28, 18.165625)
  line L23 (-30, 20.165625) -> (-30, -36.834375)
  line L24 (-28, 18.165625) -> (-28, 14.665625)
  line L25 (-28, 12.665625) -> (-28, 9.165625)
  line L26 (-28, 7.165625) -> (-28, 3.665625)
  line L27 (-28, 1.665625) -> (-28, -1.834375)
  line L28 (-28, -3.834375) -> (-28, -7.334375)
  line L29 (-28, -9.334375) -> (-28, -12.834375)
  line L30 (-28, -14.834375) -> (-28, -18.334375)
  line L31 (-28, -20.334375) -> (-28, -23.834375)
  line L32 (-28, -25.834375) -> (-28, -29.334375)
  line L33 (-28, -31.334375) -> (-28, -34.834375)
  arc A0 (-10.286978, 20.165625) -> (-10.730432, 18.165625) centre (113.517821, -8.334375) ccw
  arc A1 (-11.42568, 14.665625) -> (-11.777344, 12.665625) centre (113.517821, -8.334375) ccw
  arc A2 (-12.313925, 9.165625) -> (-12.575908, 7.165625) centre (113.517821, -8.334375) ccw
  arc A3 (-12.956992, 3.665625) -> (-13.13082, 1.665625) centre (113.517821, -8.334375) ccw
  arc A4 (-13.358609, -1.834375) -> (-13.445277, -3.834375) centre (113.517821, -8.334375) ccw
  arc A5 (-13.521064, -7.334375) -> (-13.521064, -9.334375) centre (113.517821, -8.334375) ccw
  arc A6 (-13.445277, -12.834375) -> (-13.358609, -14.834375) centre (113.517821, -8.334375) ccw
  arc A7 (-13.13082, -18.334375) -> (-12.956992, -20.334375) centre (113.517821, -8.334375) ccw
  arc A8 (-12.575908, -23.834375) -> (-12.313925, -25.834375) centre (113.517821, -8.334375) ccw
  arc A9 (-11.777344, -29.334375) -> (-11.42568, -31.334375) centre (113.517821, -8.334375) ccw
  arc A10 (-10.730432, -34.834375) -> (-10.286978, -36.834375) centre (113.517821, -8.334375) ccw
  arc A11 (146.708609, -14.834375) -> (146.795277, -12.834375) centre (19.832179, -8.334375) ccw
  arc A12 (146.48082, 1.665625) -> (146.306992, 3.665625) centre (19.832179, -8.334375) ccw
  line L34 (146.708609, -1.834375) -> (161.35, -1.834375)
  line L35 (143.636978, -36.834375) -> (163.35, -36.834375)
  line L36 (144.080432, -34.834375) -> (161.35, -34.834375)
  line L37 (146.48082, -18.334375) -> (161.35, -18.334375)
  line L38 (161.35, -20.334375) -> (161.35, -23.834375)
  line L39 (161.35, -31.334375) -> (161.35, -34.834375)
  line L40 (161.35, -25.834375) -> (161.35, -29.334375)
  line L41 (145.127344, -29.334375) -> (161.35, -29.334375)
  arc A13 (146.306992, -20.334375) -> (146.48082, -18.334375) centre (19.832179, -8.334375) ccw
  line L42 (161.35, -14.834375) -> (161.35, -18.334375)
  line L43 (144.77568, -31.334375) -> (161.35, -31.334375)
  arc A14 (144.77568, -31.334375) -> (145.127344, -29.334375) centre (19.832179, -8.334375) ccw
  line L44 (146.306992, -20.334375) -> (161.35, -20.334375)
  arc A15 (145.663925, -25.834375) -> (145.925908, -23.834375) centre (19.832179, -8.334375) ccw
  arc A16 (143.636978, -36.834375) -> (144.080432, -34.834375) centre (19.832179, -8.334375) ccw
  line L45 (145.663925, -25.834375) -> (161.35, -25.834375)
  line L46 (145.925908, -23.834375) -> (161.35, -23.834375)
  line L47 (144.080432, 18.165625) -> (161.35, 18.165625)
  line L48 (145.925908, 7.165625) -> (161.35, 7.165625)
  arc A17 (145.127344, 12.665625) -> (144.77568, 14.665625) centre (19.832179, -8.334375) ccw
  line L49 (144.77568, 14.665625) -> (161.35, 14.665625)
  line L50 (145.663925, 9.165625) -> (161.35, 9.165625)
  arc A18 (144.080432, 18.165625) -> (143.636978, 20.165625) centre (19.832179, -8.334375) ccw
  line L51 (161.35, 7.165625) -> (161.35, 3.665625)
  line L52 (146.795277, -12.834375) -> (161.35, -12.834375)
  line L53 (146.306992, 3.665625) -> (161.35, 3.665625)
  line L54 (143.636978, 20.165625) -> (163.35, 20.165625)
  line L55 (146.795277, -3.834375) -> (161.35, -3.834375)
  line L56 (161.35, 12.665625) -> (161.35, 9.165625)
  line L57 (145.127344, 12.665625) -> (161.35, 12.665625)
  arc A19 (145.925908, 7.165625) -> (145.663925, 9.165625) centre (19.832179, -8.334375) ccw
  line L58 (161.35, 1.665625) -> (161.35, -1.834375)
  line L59 (161.35, -3.834375) -> (161.35, -7.334375)
  line L60 (161.35, 18.165625) -> (161.35, 14.665625)
  line L61 (146.48082, 1.665625) -> (161.35, 1.665625)
  line L62 (146.708609, -14.834375) -> (161.35, -14.834375)
  arc A20 (146.871064, -9.334375) -> (146.871064, -7.334375) centre (19.832179, -8.334375) ccw
  line L63 (146.871064, -7.334375) -> (161.35, -7.334375)
  arc A21 (146.795277, -3.834375) -> (146.708609, -1.834375) centre (19.832179, -8.334375) ccw
  line L64 (146.871064, -9.334375) -> (161.35, -9.334375)
  line L65 (161.35, -9.334375) -> (161.35, -12.834375)
  line L66 (163.35, 20.165625) -> (163.35, -36.834375)
  point P0 (133.35, 0)
  constraint horizontal L0
  constraint horizontal L2
  constraint perpendicular L4 L23
  constraint collinear L24 L25
  constraint collinear L25 L26
  constraint collinear L26 L27
  constraint collinear L27 L28
  constraint collinear L28 L29
  constraint collinear L29 L30
  constraint collinear L30 L31
  constraint collinear L31 L32
  constraint collinear L32 L33
  constraint concentric A0 A1
  constraint concentric A1 A2
  constraint concentric A2 A3
  constraint concentric A3 A4
  constraint concentric A4 A5
  constraint concentric A5 A6
  constraint concentric A6 A7
  constraint concentric A7 A8
  constraint concentric A8 A9
  constraint concentric A9 A10
  constraint symmetric origin L1 P0
  constraint symmetric L1 A0 A18
  constraint symmetric L1 A1 A17
  constraint symmetric L1 A2 A19
  constraint symmetric L1 A3 A12
  constraint symmetric L1 A4 A21
  constraint symmetric L1 A5 A20
  constraint symmetric L1 A6 A11
  constraint symmetric L1 A7 A13
  constraint symmetric L1 A8 A15
  constraint symmetric L1 A9 A14
  constraint symmetric L1 A10 A16
sketch "sink2" plane through (0, 0, 0) normal (0, 0, 1) x (1, 0, 0)
  line L0 (-28, -20.334375) -> (-28, -23.834375)
  line L1 (-6.525, -14.834375) -> (-28, -14.834375)
  line L2 (-28, -31.334375) -> (-28, -34.834375)
  line L3 (-6.525, -7.334375) -> (-28, -7.334375)
  line L4 (-6.525, -12.834375) -> (-28, -12.834375)
  line L5 (-6.525, -20.334375) -> (-28, -20.334375)
  line L6 (-6.525, -34.834375) -> (-28, -34.834375)
  line L7 (-6.525, -23.834375) -> (-28, -23.834375)
  line L8 (-28, -9.334375) -> (-28, -12.834375)
  line L9 (-6.525, -18.334375) -> (-28, -18.334375)
  line L10 (-6.525, -3.834375) -> (-28, -3.834375)
  line L11 (-6.525, -25.834375) -> (-28, -25.834375)
  line L12 (-28, -3.834375) -> (-28, -7.334375)
  line L13 (-6.525, -36.834375) -> (-30, -36.834375)
  line L14 (-28, -25.834375) -> (-28, -29.334375)
  line L15 (-28, 12.665625) -> (-28, 9.165625)
  line L16 (-6.525, -29.334375) -> (-28, -29.334375)
  line L17 (66.675, 35.245101) -> (66.675, -62.292438)
  line L18 (-6.525, 3.665625) -> (-28, 3.665625)
  line L19 (-6.525, 20.165625) -> (-30, 20.165625)
  line L20 (-6.525, -9.334375) -> (-28, -9.334375)
  line L21 (-6.525, 1.665625) -> (-28, 1.665625)
  line L22 (-6.525, -1.834375) -> (-28, -1.834375)
  line L23 (-6.525, -31.334375) -> (-28, -31.334375)
  line L24 (-6.525, 18.165625) -> (-28, 18.165625)
  line L25 (-6.525, 7.165625) -> (-28, 7.165625)
  line L26 (-28, -14.834375) -> (-28, -18.334375)
  line L27 (-28, 1.665625) -> (-28, -1.834375)
  line L28 (-28, 18.165625) -> (-28, 14.665625)
  line L29 (-28, 7.165625) -> (-28, 3.665625)
  line L30 (-6.525, 14.665625) -> (-28, 14.665625)
  line L31 (-6.525, 9.165625) -> (-28, 9.165625)
  line L32 (-6.525, 12.665625) -> (-28, 12.665625)
  line L33 (-30, 20.165625) -> (-30, -36.834375)
  line L34 (-6.525, 20.165625) -> (-6.525, 18.165625)
  line L35 (-6.525, 14.665625) -> (-6.525, 12.665625)
  line L36 (-6.525, 9.165625) -> (-6.525, 7.165625)
  line L37 (-6.525, 3.665625) -> (-6.525, 1.665625)
  line L38 (-6.525, -1.834375) -> (-6.525, -3.834375)
  line L39 (-6.525, -7.334375) -> (-6.525, -9.334375)
  line L40 (-6.525, -12.834375) -> (-6.525, -14.834375)
  line L41 (-6.525, -18.334375) -> (-6.525, -20.334375)
  line L42 (-6.525, -23.834375) -> (-6.525, -25.834375)
  line L43 (-6.525, -29.334375) -> (-6.525, -31.334375)
  line L44 (-6.525, -34.834375) -> (-6.525, -36.834375)
  line L45 (139.875, 3.665625) -> (139.875, 1.665625)
  line L46 (139.875, 9.165625) -> (139.875, 7.165625)
  line L47 (161.35, -14.834375) -> (161.35, -18.334375)
  line L48 (139.875, -3.834375) -> (161.35, -3.834375)
  line L49 (139.875, 20.165625) -> (163.35, 20.165625)
  line L50 (139.875, 20.165625) -> (139.875, 18.165625)
  line L51 (139.875, 14.665625) -> (139.875, 12.665625)
  line L52 (161.35, 12.665625) -> (161.35, 9.165625)
  line L53 (139.875, 9.165625) -> (161.35, 9.165625)
  line L54 (139.875, -12.834375) -> (139.875, -14.834375)
  line L55 (139.875, -7.334375) -> (139.875, -9.334375)
  line L56 (161.35, 7.165625) -> (161.35, 3.665625)
  line L57 (139.875, -1.834375) -> (139.875, -3.834375)
  line L58 (139.875, -12.834375) -> (161.35, -12.834375)
  line L59 (161.35, -3.834375) -> (161.35, -7.334375)
  line L60 (161.35, 18.165625) -> (161.35, 14.665625)
  line L61 (139.875, -18.334375) -> (161.35, -18.334375)
  line L62 (139.875, -7.334375) -> (161.35, -7.334375)
  line L63 (139.875, -1.834375) -> (161.35, -1.834375)
  line L64 (139.875, -14.834375) -> (161.35, -14.834375)
  line L65 (139.875, -31.334375) -> (161.35, -31.334375)
  line L66 (139.875, -36.834375) -> (163.35, -36.834375)
  line L67 (139.875, -29.334375) -> (161.35, -29.334375)
  line L68 (139.875, 1.665625) -> (161.35, 1.665625)
  line L69 (161.35, 1.665625) -> (161.35, -1.834375)
  line L70 (161.35, -9.334375) -> (161.35, -12.834375)
  line L71 (139.875, -9.334375) -> (161.35, -9.334375)
  line L72 (163.35, 20.165625) -> (163.35, -36.834375)
  line L73 (139.875, 12.665625) -> (161.35, 12.665625)
  line L74 (139.875, 14.665625) -> (161.35, 14.665625)
  line L75 (139.875, 18.165625) -> (161.35, 18.165625)
  line L76 (139.875, 3.665625) -> (161.35, 3.665625)
  line L77 (139.875, 7.165625) -> (161.35, 7.165625)
  line L78 (161.35, -20.334375) -> (161.35, -23.834375)
  line L79 (161.35, -25.834375) -> (161.35, -29.334375)
  line L80 (139.875, -18.334375) -> (139.875, -20.334375)
  line L81 (161.35, -31.334375) -> (161.35, -34.834375)
  line L82 (139.875, -23.834375) -> (139.875, -25.834375)
  line L83 (139.875, -34.834375) -> (139.875, -36.834375)
  line L84 (139.875, -20.334375) -> (161.35, -20.334375)
  line L85 (139.875, -29.334375) -> (139.875, -31.334375)
  line L86 (139.875, -34.834375) -> (161.35, -34.834375)
  line L87 (139.875, -25.834375) -> (161.35, -25.834375)
  line L88 (139.875, -23.834375) -> (161.35, -23.834375)
  point P0 (133.35, 0)
  point P1 (133.35, 0)
  constraint horizontal L3
  constraint horizontal L20
  constraint perpendicular L13 L33
  constraint collinear L15 L28
  constraint collinear L15 L29
  constraint collinear L27 L29
  constraint collinear L12 L27
  constraint collinear L8 L12
  constraint collinear L8 L26
  constraint collinear L0 L26
  constraint collinear L0 L14
  constraint collinear L2 L14
  constraint collinear L34 L35
  constraint collinear L35 L36
  constraint collinear L36 L37
  constraint collinear L37 L38
  constraint collinear L38 L39
  constraint collinear L39 L40
  constraint collinear L40 L41
  constraint collinear L41 L42
  constraint collinear L42 L43
  constraint collinear L43 L44
  constraint symmetric origin L17 P1
fillet "Fillet1" radius 3 12 edges at (-9.525, -43.625, -1.5) (142.875, -43.625, -1.5) (142.875, 26.95625, -1.5) (-9.525, 26.95625, -1.5) (-9.525, -43.625, 4) (142.875, -43.625, 4) (142.875, 26.95625, 4) (-9.525, 26.95625, 4) (-9.525, -43.625, -7) (142.875, -43.625, -7) (142.875, 26.95625, -7) (-9.525, 26.95625, -7) on bodies 1 2 3
fillet "Fillet2" radius 2 17 edges at (137.236678, -43.625, 8) (142.422791, -43.006477, 8) (147.875, -8.334375, 8) (142.422791, 26.337727, 8) (66.675, 26.95625, 8) (-9.072791, 26.337727, 8) (-14.525, -8.334375, 8) (-9.072791, -43.006477, 8) (-3.886678, -43.625, 8) (-9.072791, -43.006477, -11) (-14.525, -8.334375, -11) (-9.072791, 26.337727, -11) (66.675, 26.95625, -11) (142.422791, 26.337727, -11) (147.875, -8.334375, -11) (142.422791, -43.006477, -11) (66.675, -43.625, -11) on bodies 2 3
extrude "Extrude8" cut sketch "sink" along normal up to surface (19 mm away) from surface at -11 contours L0 L2 L3 L4 L5 L6 L7 L8 L9 L10 L11 L12 L13 L14 L15 L16 L17 L18 L19 L20 L21 L22 L23 L24 L25 L26 L27 L28 L29 L30 L31 L32 L33 A0 A1 A2 A3 A4 A5 A6 A7 A8 A9 A10 picked at (-29.333333, -11.667708) bodies 2 3
extrude "Extrude9" cut sketch "sink" along normal up to surface (19 mm away) from surface at -11 contours A11 A12 L34 L35 L36 L37 L38 L39 L40 L41 A13 L42 L43 A14 L44 A15 A16 L45 L46 L47 L48 A17 L49 L50 A18 L51 L52 L53 L54 L55 L56 L57 A19 L58 L59 L60 L61 L62 A20 L63 A21 L64 L65 L66 picked at (162.683333, -13.501042) bodies 2 3
extrude "Extrude10" cut sketch "sink2" against normal blind 1 from surface at 8 contours L0 L1 L2 L3 L4 L5 L6 L7 L8 L9 L10 L11 L12 L13 L14 L15 L16 L18 L19 L20 L21 L22 L23 L24 L25 L26 L27 L28 L29 L30 L31 L32 L33 L34 L35 L36 L37 L38 L39 L40 L41 L42 L43 L44 picked at (-29.333333, -13.501042) bodies 2
extrude "Extrude11" cut sketch "sink2" along normal blind 1 from surface at -11 contours L0 L1 L2 L3 L4 L5 L6 L7 L8 L9 L10 L11 L12 L13 L14 L15 L16 L18 L19 L20 L21 L22 L23 L24 L25 L26 L27 L28 L29 L30 L31 L32 L33 L34 L35 L36 L37 L38 L39 L40 L41 L42 L43 L44 picked at (-29.333333, -13.501042) bodies 3
extrude "Extrude12" cut sketch "sink2" along normal blind 1 from surface at -11 contours L45 L46 L47 L48 L49 L50 L51 L52 L53 L54 L55 L56 L57 L58 L59 L60 L61 L62 L63 L64 L65 L66 L67 L68 L69 L70 L71 L72 L73 L74 L75 L76 L77 L78 L79 L80 L81 L82 L83 L84 L85 L86 L87 L88 picked at (162.683333, -4.334375) bodies 3
extrude "Extrude13" cut sketch "sink2" against normal blind 1 from surface at 8 contours L45 L46 L47 L48 L49 L50 L51 L52 L53 L54 L55 L56 L57 L58 L59 L60 L61 L62 L63 L64 L65 L66 L67 L68 L69 L70 L71 L72 L73 L74 L75 L76 L77 L78 L79 L80 L81 L82 L83 L84 L85 L86 L87 L88 picked at (162.683333, -4.334375) bodies 2
fillet "Fillet3" radius 1 6 edges at (9, 0.525, 4) (-0.525, -18.525, 4) (66.15, 0.525, 6) (48.15, 0.525, 6) (124.35, 0.525, 4) (133.875, -18.525, 4) on bodies 2
fillet "Fillet4" radius 1 4 edges at (-0.525, 21.95625, -6) (133.875, 21.95625, -6) (133.875, -38.625, -6) (-0.525, -38.625, -6) on bodies 3
sketch "usb" plane through (0, -18.525, 0) normal (0, -1, 0) x (1, 0, 0)
  line L0 (48.15, 0) -> (66.15, 0)
  line L1 (66.15, 0) -> (66.15, 8)
  line L2 (66.15, 8) -> (48.15, 8)
  line L3 (48.15, 8) -> (48.15, 0)
  line L4 (53.15, -8.5) -> (61.15, -8.5)
  line L5 (53.15, 0) -> (61.15, 0)
  line L6 (50.15, -3) -> (50.15, -5.5)
  line L7 (64.15, -3) -> (64.15, -5.5)
  arc A0 (53.15, 0) -> (50.15, -3) centre (53.15, -3) ccw
  arc A1 (50.15, -5.5) -> (53.15, -8.5) centre (53.15, -5.5) ccw
  arc A2 (61.15, -8.5) -> (64.15, -5.5) centre (61.15, -5.5) ccw
  arc A3 (64.15, -3) -> (61.15, 0) centre (61.15, -3) ccw
  line L8 (53.4, -3) -> (60.9, -3)
  line L9 (53.4, -5.5) -> (60.9, -5.5)
  line L10 (53.4, -3) -> (53.4, -5.5)
  line L11 (60.9, -3) -> (60.9, -5.5)
  dimension "d124" = 3
  constraint parallel L0 L4
  constraint perpendicular L4 L6
  constraint perpendicular L4 L7
  constraint tangent L5 A0
  constraint tangent L6 A0
  constraint tangent L4 A1
  constraint tangent L6 A1
  constraint equal A0 A1
  constraint tangent L4 A2
  constraint tangent L7 A2
  constraint equal A0 A2
  constraint tangent L5 A3
  constraint tangent L7 A3
  constraint equal A0 A3
  constraint parallel L5 L8
  constraint parallel L4 L9
  measures "d124" radius of A0
extrude "Extrude14" cut sketch "usb" against normal up to surface (3.5 mm away) from surface at -41.98125 contours L0 L4 L5 L6 L7 A0 A1 A2 A3 | L8 L9 L10 L11 picked at (58.4, -7.5) picked at (55.9, -3.833333) bodies 1
extrude "Extrude15" cut sketch "usb" against normal up to surface (3.5 mm away) from surface at -41.98125 contours L0 L4 L5 L6 L7 A0 A1 A2 A3 | L8 L9 L10 L11 picked at (58.4, -7.5) picked at (55.9, -3.833333) bodies 3